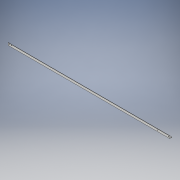
# Autodesk Inventor part: Lower Long L
Saved by Autodesk Inventor 2017 (Build 210142000, 142)
## iProperties
Created: 2018-08-22
Part Number: Lower Long L
Material: Generic
Document SubType Name: Modeling
Designer: sinner
Density: 1 g/cm^3
Appearance: Default
Author: sinner
Autodesk Inventor part; units mm, degrees
ref_plane "YZ Plane" through (0, 0, 0) normal (1, 0, 0) x (0, 1, 0)
ref_plane "XZ Plane" through (0, 0, 0) normal (0, 1, 0) x (-1, 0, 0)
ref_plane "XY Plane" through (0, 0, 0) normal (0, 0, 1) x (1, 0, 0)
sketch "Sketch1" plane through (0, 0, 0) normal (1, 0, 0) x (0, 1, 0)
  line L0 (0, 0) -> (25.4, 0)
  line L1 (25.4, 0) -> (25.4, -3.2512)
  line L2 (3.2512, -25.4) -> (0, -25.4)
  line L3 (0, -25.4) -> (0, 0)
  line L4 (25.4, -3.2512) -> (3.2512, -3.2512)
  line L5 (3.2512, -3.2512) -> (3.2512, -25.4)
  dimension "d2" = 3.2512
  dimension "d3" = 3.2512
  dimension "d4" = 25.4
  constraints: 12 end point, 4 perpendicular, 2 parallel, 1 horizontal
  measures "d2" distance between parallel lines of L0 L4
  measures "d3" distance between parallel lines of L5 L3
  measures "d4" distance of L2.end L0.start
extrude "Extrusion1" add sketch "Sketch1" along normal blind 1828.8
sketch "Sketch2" plane through (0, 0, 0) normal (0, 0, 1) x (1, 0, 0)
  line L0 (0, 0) -> (0, 25.4) projected
  line L1 (2.7844, 15.9512) -> (73.6304, 15.9512) construction
  circle A0 centre (12.7, 15.9512) radius 3.175
  circle A1 centre (38.1, 15.9512) radius 3.175
  line L2 (0, 25.4) -> (1828.8, 25.4) projected
  line L3 (0, 0) -> (1828.8, 0) projected
  dimension "d7" = 6.35
  dimension "d8" = 12.7
  dimension "d9" = 38.1
  dimension "d20" = 15.9512
  constraints: 2 centre point, 2 end point, 2 point on line, 1 equal radius, 1 parallel
  measures "d7" diameter of A1
  measures "d8" distance from line of L0 A0.centre
  measures "d9" distance from line of L0 A1.centre
  measures "d20" distance between parallel lines of L3 L1
extrude "Extrusion2" cut sketch "Sketch2" against normal blind 1828.8
sketch "Sketch3" plane through (0, 0, -25.4) normal (0, -1, 0) x (1, 0, 0)
  line L0 (1.3644, 9.4488) -> (86.9618, 9.4488) construction
  circle A0 centre (266.7, 9.4488) radius 3.175
  circle A1 centre (292.1, 9.4488) radius 3.175
  line L1 (0, 25.4) -> (1828.8, 25.4) projected
  line L2 (0, 0) -> (0, 25.4) projected
  dimension "d12" = 6.35
  dimension "d17" = 15.9512
  dimension "d18" = 266.7
  dimension "d19" = 292.1
  constraints: 2 centre point, 2 end point, 2 point on line, 1 equal radius, 1 parallel
  measures "d12" diameter of A1
  measures "d17" distance between parallel lines of L1 L0
  measures "d18" distance from line of L2 A0.centre
  measures "d19" distance from line of L2 A1.centre
extrude "Extrusion3" cut sketch "Sketch3" against normal blind 1828.8
sketch "Sketch4" plane through (0, 0, 0) normal (0, 0, 1) x (1, 0, 0)
  line L0 (1828.8, 25.4) -> (1828.8, 0) projected
  line L1 (1828.8, 12.7) -> (1190.8061, 12.7) construction
  circle A0 centre (1816.1, 12.7) radius 3.175
  circle A1 centre (1689.1, 12.7) radius 3.175
  point P0 (0, 0)
  dimension "d21" = 6.35
  dimension "d22" = 12.7
  dimension "d23" = 139.7
  constraints: 2 centre point, 2 end point, 2 point on line, 1 equal radius, 1 horizontal, 1 midpoint
  measures "d21" diameter of A0
  measures "d22" distance from line of L0 A0.centre
  measures "d23" distance from line of L0 A1.centre
extrude "Extrusion4" cut sketch "Sketch4" against normal blind 1828.8
sketch "Sketch5" plane through (0, 0, -25.4) normal (0, -1, 0) x (1, 0, 0)
  line L0 (1828.8, 0) -> (1828.8, 22.1488) projected
  line L1 (1828.8, 11.0744) -> (1744.1467, 11.0744) construction
  circle A0 centre (1689.1, 11.0744) radius 3.175
  circle A1 centre (1816.1, 11.0744) radius 3.175
  point P0 (0, 25.4)
  dimension "d26" = 6.35
  dimension "d27" = 12.7
  dimension "d28" = 139.7
  constraints: 2 centre point, 2 end point, 2 point on line, 1 equal radius, 1 horizontal, 1 midpoint
  measures "d26" diameter of A1
  measures "d27" distance from line of L0 A1.centre
  measures "d28" distance from line of L0 A0.centre
extrude "Extrusion5" cut sketch "Sketch5" against normal blind 1828.8
body "Solid1"
